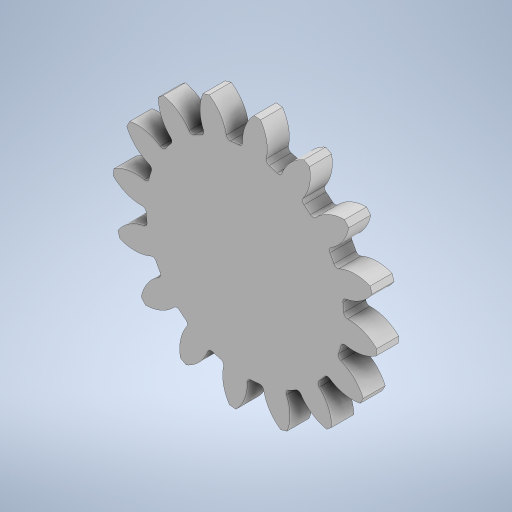
# Autodesk Inventor part: 16P_Recto
Saved by Autodesk Inventor 2023 (Build 270158030, 158C)
## iProperties
Created: 2022-05-28
Part Number: 16P_Recto
Material: Genérico
Document SubType Name: Modeling
Designer: isaac
Density: 1 g/cm^3
Appearance: Valor por defecto
Author: isaac
Autodesk Inventor part; units mm, degrees
ref_plane "YZ Plane" through (0, 0, 0) normal (1, 0, 0) x (0, 1, 0)
ref_plane "XZ Plane" through (0, 0, 0) normal (0, 1, 0) x (-1, 0, 0)
ref_plane "XY Plane" through (0, 0, 0) normal (0, 0, 1) x (1, 0, 0)
sketch "Boceto1" plane through (0, 0, 0) normal (0, 0, 1) x (1, 0, 0)
  arc A0 (178.7516, -21.1631) -> (179.5772, -12.3304) centre (0, 0) ccw
  circle A1 centre (0, 0) radius 135
  arc A2 (179.5772, -12.3304) -> (134.9681, 2.9346) centre (141.2836, -51.423) ccw
  arc A3 (132.0863, -27.8965) -> (178.7516, -21.1631) centre (148.3661, 24.3491) ccw
  arc A4 (173.2437, 48.8532) -> (170.6263, 57.3294) centre (0, 0) ccw
  arc A5 (170.6263, 57.3294) -> (123.5713, 54.3612) centre (150.2077, 6.5582) ccw
  arc A6 (132.7073, 24.7742) -> (173.2437, 48.8532) centre (127.7544, 79.2728) ccw
  arc A7 (141.361, 111.4319) -> (135.6992, 118.2613) centre (0, 0) ccw
  arc A8 (135.6992, 118.2613) -> (93.3618, 97.5119) centre (136.2641, 63.541) ccw
  arc A9 (113.1249, 73.6733) -> (141.361, 111.4319) centre (87.6933, 122.128) ccw
  arc A10 (87.9574, 157.0462) -> (80.113, 161.189) centre (0, 0) ccw
  arc A11 (80.113, 161.189) -> (48.9389, 125.8173) centre (101.5755, 110.8503) ccw
  arc A12 (76.3202, 111.3563) -> (87.9574, 157.0462) centre (34.2816, 146.3904) ccw
  arc A13 (21.1631, 178.7516) -> (12.3304, 179.5772) centre (0, 0) ccw
  arc A14 (12.3304, 179.5772) -> (-2.9346, 134.9681) centre (51.423, 141.2836) ccw
  arc A15 (27.8965, 132.0863) -> (21.1631, 178.7516) centre (-24.3491, 148.3661) ccw
  arc A16 (-48.8532, 173.2437) -> (-57.3294, 170.6263) centre (0, 0) ccw
  arc A17 (-57.3294, 170.6263) -> (-54.3612, 123.5713) centre (-6.5582, 150.2077) ccw
  arc A18 (-24.7742, 132.7073) -> (-48.8532, 173.2437) centre (-79.2728, 127.7544) ccw
  arc A19 (-111.4319, 141.361) -> (-118.2613, 135.6992) centre (0, 0) ccw
  arc A20 (-118.2613, 135.6992) -> (-97.5119, 93.3618) centre (-63.541, 136.2641) ccw
  arc A21 (-73.6733, 113.1249) -> (-111.4319, 141.361) centre (-122.128, 87.6933) ccw
  arc A22 (-157.0462, 87.9574) -> (-161.189, 80.113) centre (0, 0) ccw
  arc A23 (-161.189, 80.113) -> (-125.8173, 48.9389) centre (-110.8503, 101.5755) ccw
  arc A24 (-111.3563, 76.3202) -> (-157.0462, 87.9574) centre (-146.3904, 34.2816) ccw
  arc A25 (-178.7516, 21.1631) -> (-179.5772, 12.3304) centre (0, 0) ccw
  arc A26 (-179.5772, 12.3304) -> (-134.9681, -2.9346) centre (-141.2836, 51.423) ccw
  arc A27 (-132.0863, 27.8965) -> (-178.7516, 21.1631) centre (-148.3661, -24.3491) ccw
  arc A28 (-173.2437, -48.8532) -> (-170.6263, -57.3294) centre (0, 0) ccw
  arc A29 (-170.6263, -57.3294) -> (-123.5713, -54.3612) centre (-150.2077, -6.5582) ccw
  arc A30 (-132.7073, -24.7742) -> (-173.2437, -48.8532) centre (-127.7544, -79.2728) ccw
  arc A31 (-141.361, -111.4319) -> (-135.6992, -118.2613) centre (0, 0) ccw
  arc A32 (-135.6992, -118.2613) -> (-93.3618, -97.5119) centre (-136.2641, -63.541) ccw
  arc A33 (-113.1249, -73.6733) -> (-141.361, -111.4319) centre (-87.6933, -122.128) ccw
  arc A34 (-87.9574, -157.0462) -> (-80.113, -161.189) centre (0, 0) ccw
  arc A35 (-80.113, -161.189) -> (-48.9389, -125.8173) centre (-101.5755, -110.8503) ccw
  arc A36 (-76.3202, -111.3563) -> (-87.9574, -157.0462) centre (-34.2816, -146.3904) ccw
  arc A37 (-21.1631, -178.7516) -> (-12.3304, -179.5772) centre (0, 0) ccw
  arc A38 (-12.3304, -179.5772) -> (2.9346, -134.9681) centre (-51.423, -141.2836) ccw
  arc A39 (-27.8965, -132.0863) -> (-21.1631, -178.7516) centre (24.3491, -148.3661) ccw
  arc A40 (48.8532, -173.2437) -> (57.3294, -170.6263) centre (0, 0) ccw
  arc A41 (57.3294, -170.6263) -> (54.3612, -123.5713) centre (6.5582, -150.2077) ccw
  arc A42 (24.7742, -132.7073) -> (48.8532, -173.2437) centre (79.2728, -127.7544) ccw
  arc A43 (111.4319, -141.361) -> (118.2613, -135.6992) centre (0, 0) ccw
  arc A44 (118.2613, -135.6992) -> (97.5119, -93.3618) centre (63.541, -136.2641) ccw
  arc A45 (73.6733, -113.1249) -> (111.4319, -141.361) centre (122.128, -87.6933) ccw
  arc A46 (157.0462, -87.9574) -> (161.189, -80.113) centre (0, 0) ccw
  arc A47 (161.189, -80.113) -> (125.8173, -48.9389) centre (110.8503, -101.5755) ccw
  arc A48 (111.3563, -76.3202) -> (157.0462, -87.9574) centre (146.3904, -34.2816) ccw
  point P0 (97.5119, -93.3618)
  point P1 (125.8173, -48.9389)
  point P2 (132.0863, -27.8965)
  point P3 (132.7073, 24.7742)
  point P4 (123.5713, 54.3612)
  point P5 (48.9389, 125.8173)
  point P6 (27.8965, 132.0863)
  point P7 (-2.9346, 134.9681)
  point P8 (-24.7742, 132.7073)
  point P9 (-54.3612, 123.5713)
  point P10 (-125.8173, 48.9389)
  point P11 (-132.0863, 27.8965)
  point P12 (-134.9681, -2.9346)
  point P13 (-113.1249, -73.6733)
  point P14 (-48.9389, -125.8173)
  point P15 (2.9346, -134.9681)
  point P16 (24.7742, -132.7073)
  point P17 (54.3612, -123.5713)
  point P18 (73.6733, -113.1249)
  dimension "d8" = 360
  constraints: 96 point on circle, 48 centre point, 3 coincident, 162 other
extrude "Extrusión1" add sketch "Boceto1" along normal blind 30
fillet "Empalme1" radius 5.235 2 edges at (76.3202, 111.3563, 15) (93.3618, 97.5119, 15)
pattern_circular "Patrón circular1" count 16 over 360 about axis through (0, 0, 0) along (0, 0, 1) of "Empalme1"
